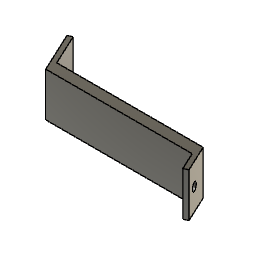
landing-gear-leg (Autodesk Fusion 360 design; units mm, degrees)
Autodesk Fusion 360 part; units mm, degrees
sketch "Sketch1" plane through (0, 0, 0) normal (0, 0, 1) x (1, 0, 0)
  line L0 (55.4833, 22.0753) -> (95.4833, 22.0753)
  line L1 (95.4833, 22.0753) -> (95.4833, 19.0753)
  line L2 (95.4833, 19.0753) -> (55.4833, 19.0753)
  line L3 (55.4833, 19.0753) -> (55.4833, 22.0753)
  line L4 (95.4833, 22.0753) -> (98.8643, 14.8248)
  line L5 (98.8643, 14.8248) -> (97.7152, 14.289)
  line L6 (97.7152, 14.289) -> (95.4833, 19.0753)
  line L7 (55.4833, 19.0753) -> (50.4119, 29.951)
  line L8 (50.4119, 29.951) -> (51.561, 30.4868)
  line L9 (55.4833, 22.0753) -> (51.561, 30.4868)
  dimension "d2" = 3
  dimension "d3" = 40
  dimension "d5" = 115
  dimension "d8" = 115
  dimension "d9" = 115
  dimension "d10" = 115
  dimension "d12" = 8
  dimension "d13" = 12
  constraint horizontal L0
  constraint vertical L1
  constraint horizontal L2
  constraint vertical L3
  constraint perpendicular L5 L6
  constraint perpendicular L8 L9
  measures "d2" distance of L0.start L2.end
  measures "d3" distance of L0.start L0.end
  measures "d5" angle of L0 L4
  measures "d8" angle of L2 L7
  measures "d9" angle of L2 L6
  measures "d10" angle of L0 L9
  measures "d12" distance of L0.end L4.end
  measures "d13" distance of L2.end L7.end
extrude "Extrude1" add sketch "Sketch1" along normal blind 12
sketch "Sketch2" plane through (86.8847, 40.515, 0) normal (0.906308, 0.422618, 0) x (-0.422618, 0.906308, 0)
  line L0 (-28.346, 0) -> (-20.346, 0)
  line L1 (-20.346, 0) -> (-20.346, 12)
  line L2 (-20.346, 12) -> (-28.346, 12)
  line L3 (-28.346, 12) -> (-28.346, 0)
  line L4 (-25.346, 12) -> (-25.346, 0) construction
  line L5 (-20.346, 6) -> (-28.346, 6) construction
  circle A0 centre (-25.346, 6) radius 1.1
  dimension "d17" = 2.2
  dimension "d23" = 3
  constraint perpendicular L2 L4
  constraint midpoint L1 L5.start
  constraint midpoint L3 L5.end
  constraint midpoint L4 A0.centre
  constraint coincident L2 L4.start
  constraint coincident L0 L4.end
  measures "d17" diameter of A0
  measures "d23" distance of L3 L4
extrude "Extrude2" cut sketch "Sketch2" against normal up to surface (1.2679 mm away) contours A0
sketch "Sketch4" plane through (54.029, 25.1941, 0) normal (0.906308, 0.422618, 0) x (-0.422618, 0.906308, 0)
  line L0 (-3.4413, 0) -> (5.8398, 0)
  line L1 (5.8398, 0) -> (5.8398, 12)
  line L2 (5.8398, 12) -> (-3.4413, 12)
  line L3 (-3.4413, 12) -> (-3.4413, 0)
  line L4 (1.1993, 12) -> (1.1993, 0) construction
  line L5 (5.8398, 6) -> (-3.4413, 6) construction
  circle A0 centre (1.1993, 6) radius 1
  dimension "d24" = 2
  constraint midpoint L2 L4.start
  constraint midpoint L0 L4.end
  constraint midpoint L1 L5.start
  constraint midpoint L3 L5.end
  constraint midpoint L4 A0.centre
  measures "d24" diameter of A0
extrude "Extrude3" cut sketch "Sketch4" against normal up to surface (1.2679 mm away) contours A0
equation "thickness = 3 mm"
equation "d2 = thickness"
equation "d3 = height"
equation "height = 40 mm"
equation "skid_length = 30 mm"
